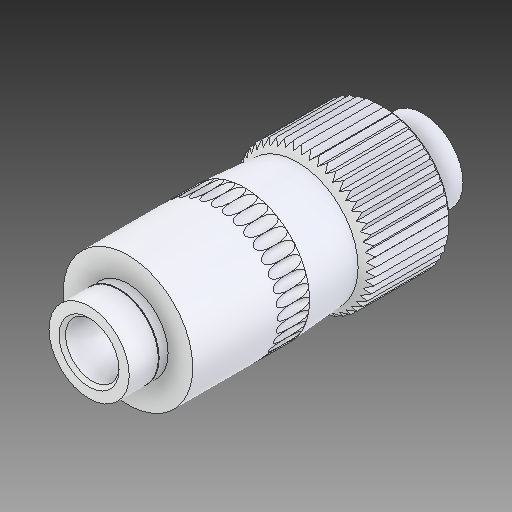
# Autodesk Inventor part: hobbed wheel
Saved by Autodesk Inventor 2018 (Build 220112000, 112)
## iProperties
Created: 2016-06-23
Part Number: hobbed wheel
Material: Generic
Document SubType Name: Modeling
Designer: Ben
Density: 1 g/cm^3
Appearance: Default
Author: Ben
Autodesk Inventor part; units mm, degrees
ref_plane "YZ Plane" through (0, 0, 0) normal (1, 0, 0) x (0, 1, 0)
sketch "Sketch1" plane through (0, 0, 0) normal (1, 0, 0) x (0, 1, 0)
  line L0 (1.65, 0) -> (1.65, 20.6)
  line L1 (1.65, 20.6) -> (2.475, 20.6)
  line L2 (2.475, 20.6) -> (2.475, 18.8)
  line L3 (2.475, 18.8) -> (2.425, 18.8)
  line L4 (2.425, 18.8) -> (2.425, 18.75)
  line L5 (2.425, 18.75) -> (2.475, 18.75)
  line L6 (2.475, 18.75) -> (2.475, 18.2)
  line L7 (2.475, 18.2) -> (4, 18.2)
  line L8 (4, 18.2) -> (4, 11)
  line L9 (4, 11) -> (3.75, 7.75)
  line L10 (3.75, 7.75) -> (4.3, 7.2)
  line L11 (4.3, 7.2) -> (4.3, 2.7)
  line L12 (2.475, 2.4) -> (2.475, 1.85)
  line L13 (2.475, 1.85) -> (2.425, 1.85)
  line L14 (2.425, 1.85) -> (2.425, 1.8)
  line L15 (2.425, 1.8) -> (2.475, 1.8)
  line L16 (2.475, 1.8) -> (2.475, 0)
  line L17 (2.475, 0) -> (1.65, 0)
  line L18 (0, 0) -> (0, 22.9786) construction
  line L19 (2.475, 2.4) -> (4, 2.4)
  line L20 (4, 2.4) -> (4.3, 2.7)
  line L21 (4.3, 4.95) -> (6.55, 4.95) construction
  dimension "d0" = 3.3
  dimension "d1" = 4.95
  dimension "d3" = 0.05
  dimension "d4" = 0.05
  dimension "d5" = 1.8
  dimension "d6" = 8.6
  dimension "d7" = 135
  dimension "d8" = 2.4
  dimension "d9" = 8
  dimension "d10" = 4.5
  dimension "d11" = 135
  dimension "d12" = 7.5
  dimension "d13" = 0.05
  dimension "d14" = 0.05
  dimension "d16" = 20.6
  dimension "d17" = 1.8
  dimension "d19" = 8
  dimension "d20" = 2.4
  dimension "d22" = 7.2
  dimension "d49" = 4.95
  constraints: 44 end point, 11 perpendicular, 5 point on line, 2 horizontal, 2 parallel, 2 vertical, 1 collinear, 1 midpoint
  measures "d0" diameter of L0 L18
  measures "d1" diameter of L2 L18
  measures "d3" distance between parallel lines of L16 L14
  measures "d4" distance between parallel lines of L13 L15
  measures "d5" distance of L15.end L16.end
  measures "d6" diameter of L11 L18
  measures "d7" angle of L19 L20
  measures "d8" distance between parallel lines of L17 L19
  measures "d9" diameter of L19.end L18
  measures "d10" distance of L10.end L11.end
  measures "d11" angle of L11 L10
  measures "d12" diameter of L9.end L18
  measures "d13" distance between parallel lines of L5 L3
  measures "d14" distance between parallel lines of L2 L4
  measures "d16" distance between parallel lines of L17 L1
  measures "d17" distance between parallel lines of L3 L1
  measures "d19" diameter of L8 L18
  measures "d20" distance between parallel lines of L1 L7
  measures "d22" distance from line of L7 L8.end
  measures "d49" distance between parallel lines of L17 L21
revolve "Revolution1" add sketch "Sketch1" angle 360 about axis through (0, 0, 0) along (0, 0, 1)
sketch "Sketch2" plane through (0, 0, 2.4) normal (0, 0, -1) x (-1, 0, 0)
  circle A0 centre (0, 0) radius 4.3 projected
  line L0 (0, 0) -> (0, -4.3) construction
  line L1 (0, 0) -> (-0.27, -4.2915) construction
  circle A1 centre (0, 0) radius 4.3 projected
  line L2 (-0.27, -4.2915) -> (0, -4)
  line L3 (0, -4) -> (0.27, -4.2915)
  arc A2 (-0.27, -4.2915) -> (0.27, -4.2915) centre (0, 0) ccw
  dimension "d23" = 8.6
  dimension "d24" = 3.6
  dimension "d26" = 4
  constraints: 8 end point, 7 point on circle, 1 centre point, 1 coincident, 1 point on line, 1 vertical, 1 other
  measures "d23" diameter of A0
  measures "d24" angle of L1 L0
  measures "d26" distance of point (0, 0) L2.end
extrude "Extrusion1" cut sketch "Sketch2" against normal blind 6 contours L2 L3 A0 picked at (-0.12, -4.1969)
pattern_circular "Circular Pattern1" count 50 over 360 about axis through (0, 0, -10) along (0, 0, 1) of "Extrusion1"
ref_plane "Work Plane1" through (0, 0, 12) normal (0, 0, 1) x (1, 0, 0)
sketch "Sketch3" plane through (0, 0, 12) normal (0, 0, 1) x (1, 0, 0)
  circle A0 centre (0, 0) radius 4 construction
  line L0 (0, 0) -> (0, 5.8939) construction
  circle A1 centre (0, 4.1) radius 0.3672
  line L1 (2.82, 5.75) -> (-2.3672, 5.75) construction
  arc A2 (0.3486, 3.9848) -> (-0.3486, 3.9848) centre (0, 0) ccw
  dimension "d33" = 5.75
  dimension "d35" = 4.1
  dimension "d36" = 8
  dimension "d37" = 0.6981
  constraints: 6 point on circle, 4 end point, 2 centre point, 1 coincident, 1 horizontal, 1 point on line, 1 vertical
  measures "d33" distance from line of point (0, 0) L1
  measures "d35" distance of point (0, 0) A1.centre
  measures "d36" diameter of A0
revolve "Revolution2" cut sketch "Sketch3" angle 360 about axis through (2.82, 5.75, 12) along (-1, 0, 0)
pattern_circular "Circular Pattern2" count 36 over 360 about axis through (0, 0, -10) along (0, 0, 1) of "Revolution2"
chamfer "Chamfer1" distance 0.2 angle 45 2 edges at (0, -1.65, 20.6) (0, -1.65, 0)
ref_plane "Work Plane2" through (0, 0, 4.95) normal (0, 0, -1) x (-1, 0, 0)
equation "\"d13\" = d4"
equation "\"d14\" = d3"
equation "\"d17\" = d5"
equation "\"d20\" = d8"
equation "\"d37\" = 0.0872664 * d36"
equation "\"d50\" = -d49"
body "Solid1"
